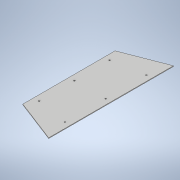
# Autodesk Inventor part: angledfloorfit2
Saved by Autodesk Inventor 2021 (Build 250183000, 183)
## iProperties
Created: 2020-10-26
Part Number: angledfloorfit2
Material: Generic
Document SubType Name: Modeling
Designer: mackeycj
Density: 1 g/cm^3
Appearance: Default
Author: mackeycj
Autodesk Inventor part; units mm, degrees
ref_plane "YZ Plane" through (0, 0, 0) normal (1, 0, 0) x (0, 1, 0)
ref_plane "XZ Plane" through (0, 0, 0) normal (0, 1, 0) x (-1, 0, 0)
ref_plane "XY Plane" through (0, 0, 0) normal (0, 0, 1) x (1, 0, 0)
sketch "Sketch1" plane through (0, 0, 0) normal (0, 1, 0) x (-1, 0, 0)
  line L0 (0, 0) -> (0, 292.1)
  line L1 (0, 0) -> (0, -292.1)
  line L2 (0, 0) -> (197.104, 0)
  line L3 (197.104, 0) -> (197.104, 215.9)
  line L4 (197.104, 0) -> (197.104, -215.9)
  line L5 (197.104, -215.9) -> (0, -292.1)
  line L6 (197.104, 215.9) -> (0, 292.1)
  line L7 (197.104, 215.9) -> (197.104, 165.1)
  line L8 (197.104, 165.1) -> (171.704, 165.1)
  circle A0 centre (171.704, 165.1) radius 3.175
  line L9 (0, 292.1) -> (0, 190.5)
  line L10 (0, -292.1) -> (0, -190.5)
  line L11 (0, -190.5) -> (25.4, -190.5)
  line L12 (0, 190.5) -> (25.4, 190.5)
  line L13 (197.104, 0) -> (171.704, 0)
  line L14 (0, 0) -> (25.4, 0)
  circle A1 centre (171.704, 0) radius 3.175
  circle A2 centre (25.4, 0) radius 3.175
  line L15 (197.104, -215.9) -> (197.104, -165.1)
  line L16 (197.104, -165.1) -> (171.704, -165.1)
  circle A3 centre (171.704, -165.1) radius 3.175
  circle A4 centre (25.4, -190.5) radius 3.175
  circle A5 centre (25.4, 190.5) radius 3.175
  dimension "d0" = 292.1
  dimension "d1" = 292.1
  dimension "d2" = 197.104
  dimension "d3" = 215.9
  dimension "d4" = 215.9
  dimension "d7" = 50.8
  dimension "d8" = 25.4
  dimension "d9" = 6.35
  dimension "d10" = 101.6
  dimension "d11" = 101.6
  dimension "d12" = 25.4
  dimension "d13" = 25.4
  dimension "d14" = 25.4
  dimension "d15" = 25.4
  dimension "d16" = 6.35
  dimension "d17" = 6.35
  dimension "d18" = 50.8
  dimension "d19" = 25.4
  dimension "d20" = 6.35
  dimension "d21" = 6.35
  dimension "d22" = 6.35
  constraints: 34 end point, 6 centre point, 6 coincident, 6 point on line, 5 perpendicular, 3 vertical, 1 horizontal
  measures "d0" distance of L0.start L0.end
  measures "d1" distance of L0.start L1.end
  measures "d2" distance of L0.start L2.end
  measures "d3" distance of L2.end L3.end
  measures "d4" distance of L2.end L4.end
  measures "d7" distance of L3.end L7.end
  measures "d8" distance of L7.end L8.end
  measures "d9" diameter of A0
  measures "d10" distance of L0.end L9.end
  measures "d11" distance of L1.end L10.end
  measures "d12" distance of L10.end L11.end
  measures "d13" distance of L9.end L12.end
  measures "d14" distance of L2.end L13.end
  measures "d15" distance of L0.start L14.end
  measures "d16" diameter of A1
  measures "d17" diameter of A2
  measures "d18" distance of L4.end L15.end
  measures "d19" distance of L15.end L16.end
  measures "d20" diameter of A3
  measures "d21" diameter of A4
  measures "d22" diameter of A5
extrude "Extrusion1" add sketch "Sketch1" along normal blind 3.175 contours L2 A2 A1 L4 L5 L1 | L0 L6 L3 L2 A1 A2
body "Solid1"
